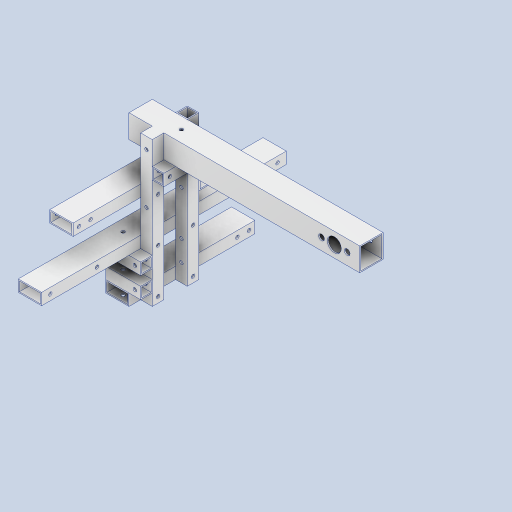
# Autodesk Inventor part: ballhand-v2-ASP-Base
Saved by Autodesk Inventor 2024 (Build 280153000, 153)
## iProperties
Created: 2024-03-16
Part Number: ballhand-v2-ASP-Base
Material: アルミニウム 6061
Document SubType Name: Modeling
Designer: haruy
Density: 2.7 g/cm^3
Appearance: アルミニウム - フラット
Author: haruy
Autodesk Inventor part; units mm, degrees
derived "ballhand-v2-Sketch-Base.ipt"
sketch "横から" plane through (0, 0, 0) normal (0, 0, 1) x (1, 0, 0)
  circle A0 centre (0, 0) radius 95
  line L0 (-321.6558, -95) -> (545.18, -95)
  line L1 (95, 81) -> (293, 81)
  line L2 (293, 81) -> (293, 61)
  line L3 (293, 61) -> (95, 61)
  line L4 (95, 61) -> (95, 81)
  line L5 (-52.5, 46.5) -> (145, 46.5)
  line L6 (145, 46.5) -> (145, 36.5)
  line L7 (145, 36.5) -> (-52.5, 36.5)
  line L8 (-52.5, 36.5) -> (-52.5, 46.5)
  line L9 (-52.5, -36.5) -> (145, -36.5)
  line L10 (145, -36.5) -> (145, -46.5)
  line L11 (145, -46.5) -> (-52.5, -46.5)
  line L12 (-52.5, -46.5) -> (-52.5, -36.5)
  line L13 (-50.5, 46.5) -> (-44.5, 46.5)
  line L14 (-44.5, 46.5) -> (-44.5, -46.5)
  line L15 (-44.5, -46.5) -> (-50.5, -46.5)
  line L16 (-50.5, -46.5) -> (-50.5, 46.5)
  line L17 (95, 5) -> (115, 5)
  line L18 (115, 5) -> (115, -5)
  line L19 (115, -5) -> (95, -5)
  line L20 (95, -5) -> (95, 5)
  line L21 (115, 4.5) -> (117.2, 4.5)
  line L22 (117.2, 4.5) -> (117.2, -4.5)
  line L23 (117.2, -4.5) -> (115, -4.5)
  line L24 (115, -4.5) -> (115, 4.5)
  line L25 (117.2, 10) -> (125, 10)
  line L26 (125, 10) -> (125, -10)
  line L27 (125, -10) -> (117.2, -10)
  line L28 (117.2, -10) -> (117.2, 10)
  line L29 (125, 46.5) -> (135, 46.5)
  line L30 (135, 46.5) -> (135, -46.5)
  line L31 (135, -46.5) -> (125, -46.5)
  line L32 (125, -46.5) -> (125, 46.5)
  line L33 (135, 36.5) -> (145, 36.5)
  line L34 (145, 36.5) -> (145, 26.5)
  line L35 (145, 26.5) -> (135, 26.5)
  line L36 (135, 26.5) -> (135, 36.5)
  line L37 (135, -36.5) -> (145, -36.5)
  line L38 (145, -36.5) -> (145, -26.5)
  line L39 (145, -26.5) -> (135, -26.5)
  line L40 (135, -26.5) -> (135, -36.5)
  line L41 (95, 33) -> (115, 33)
  line L42 (115, 33) -> (115, 43)
  line L43 (115, 43) -> (95, 43)
  line L44 (95, 43) -> (95, 33)
  line L45 (0, 0) -> (115, 0)
  line L46 (95, -33) -> (115, -33)
  line L47 (115, -43) -> (95, -43)
  line L48 (95, -43) -> (95, -33)
  line L49 (115, -33) -> (115, -43)
  line L50 (115, 81) -> (125, 81)
  line L51 (125, 81) -> (125, -43)
  line L52 (125, -43) -> (115, -43)
  line L53 (115, -43) -> (115, 81)
  circle A1 centre (105, 19) radius 2.5
  line L54 (125, 61) -> (135, 61)
  line L55 (135, 61) -> (135, 51)
  line L56 (135, 51) -> (125, 51)
  line L57 (125, 51) -> (125, 61)
  line L58 (95, 33) -> (125, 33)
  line L59 (125, 33) -> (125, 23)
  line L60 (125, 23) -> (95, 23)
  line L61 (95, 23) -> (95, 33)
  line L62 (95, -33) -> (125, -33)
  line L63 (125, -33) -> (125, -23)
  line L64 (125, -23) -> (95, -23)
  line L65 (95, -23) -> (95, -33)
  line L66 (95, -5) -> (125, -5)
  line L67 (125, -5) -> (125, -15)
  line L68 (125, -15) -> (95, -15)
  line L69 (95, -15) -> (95, -5)
  point P0 (120, 71)
  point P1 (271.25, 71)
  point P2 (260.25, 71)
  point P3 (282.25, 71)
  point P4 (120, 81)
  point P5 (120, 28)
  point P6 (120, -10)
  point P7 (120, -28)
  dimension "d1" = 10
  dimension "d2" = 10
  dimension "d3" = 30
  dimension "d4" = 10
  dimension "d7" = 30
  dimension "d8" = 10
  dimension "d9" = 30
  dimension "d10" = 10
  dimension "d11" = 21.75
  dimension "d12" = 11
  dimension "d13" = 11
  dimension "d14" = 10
  dimension "d15" = 10
  dimension "d16" = 10
  dimension "d17" = 5
  dimension "d18" = 10
  dimension "d19" = 5
  dimension "d20" = 5
  dimension "d21" = 5
  dimension "d22" = 5
  dimension "d23" = 5
  dimension "d24" = 5
  measures "d1" distance of L55.end L56.end
  measures "d2" distance of L54.end L55.end
  measures "d3" distance of L59.end L60.end
  measures "d4" distance of L58.end L59.end
  measures "d7" distance of L64.end L63.end
  measures "d8" distance of L63.end L62.end
  measures "d9" distance of L67.end L68.end
  measures "d10" distance of L66.end L67.end
  measures "d11" distance from line of point (271.25, 71) L2
  measures "d12" distance of point (271.25, 71) point (282.25, 71)
  measures "d13" distance of point (260.25, 71) point (271.25, 71)
  measures "d14" distance from line of point (260.25, 71) L1
  measures "d15" distance from line of point (271.25, 71) L1
  measures "d16" distance from line of point (282.25, 71) L1
  measures "d17" distance from line of L53 point (120, 71)
  measures "d18" distance of point (120, 71) point (120, 81)
  measures "d19" distance from line of point (120, 28) L32
  measures "d20" distance from line of L58 point (120, 28)
  measures "d21" distance from line of point (120, -10) L67
  measures "d22" distance from line of L66 point (120, -10)
  measures "d23" distance from line of point (120, -28) L51
  measures "d24" distance from line of L64 point (120, -28)
extrude "押し出し1" add sketch "横から" against normal blind 20 contours L53 L1 L51 L3 | L3 L4 L1 L53 | L51 L1 L2 L3
extrude "押し出し2" add sketch "横から" along normal blind 10 contours L18 L21 L22 L23 | L66 L28 L27 L32 L68 L53 | L18 L23 L28 L66 | L53 L60 L32 L25 L28 L21 L18 | L53 L3 L51 L5 | L5 L32 L7 L42 L53 | L7 L32 L58 L42 | L49 L62 L32 L9 | L9 L32 L52 L49 | L68 L32 L64 L53 | L66 L26 L27 L28 | L28 L22 L25 L26 L66 | L53 L58 L32 L60 | L53 L1 L51 L3 | L53 L64 L32 L62
ref_plane "作業平面1" through (293, 61, -20) normal (0, 0, -1) x (-1, 0, 0)
extrude "押し出し3" add sketch "横から" against normal blind 10 from surface at -20 separate body contours L18 L21 L22 L23 | L66 L28 L27 L32 L68 L53 | L18 L23 L28 L66 | L53 L60 L32 L25 L28 L21 L18 | L53 L3 L51 L5 | L5 L32 L7 L42 L53 | L7 L32 L58 L42 | L49 L62 L32 L9 | L9 L32 L52 L49 | L68 L32 L64 L53 | L66 L26 L27 L28 | L28 L22 L25 L26 L66 | L53 L58 L32 L60 | L53 L1 L51 L3 | L53 L64 L32 L62
extrude "押し出し4" add sketch "横から" along normal blind 10 and the other way blind 30 separate body contours L51 L3 L55 L56
extrude "押し出し5" add sketch "横から" along normal blind 95 and the other way blind 115 separate body contours L45 L18 L19 L20 | L20 L17 L18 L45
extrude "押し出し6" add sketch "横から" along normal blind 68 and the other way blind 40 separate body contours L44 L43 L42 L7 | L7 L42 L41 L44
extrude "押し出し7" add sketch "横から" along normal blind 20 and the other way blind 88 separate body contours L48 L46 L49 L9 | L9 L49 L47 L48
ref_plane "作業平面2" through (125, -43, -30) normal (0, 0, -1) x (-1, 0, 0)
extrude "押し出し8" add sketch "横から" against normal blind 10 from surface at -30 separate body contours L41 L53 L60 L61 | L53 L58 L32 L60
ref_plane "作業平面3" through (115, -43, 10) normal (0, 0, 1) x (1, 0, 0)
extrude "押し出し9" add sketch "横から" along normal blind 10 from surface at 10 separate body contours L65 L64 L53 L46 | L53 L64 L32 L62
extrude "押し出し10" add sketch "横から" along normal blind 10 from surface at 10 separate body contours L19 L53 L68 L69 | L66 L28 L27 L32 L68 L53 | L66 L26 L27 L28
shell "シェル1" thickness 1 removed faces 20 at (95, 74.3333, -13.3333) at (293, 67.6667, -6.6667) at (121.6667, 81, -23.3333) at (131.6667, 54.3333, -30) at (131.6667, 54.3333, 10) at (118.3333, -43, 3.3333) at (118.3333, -43, -23.3333) at (101.6667, -39.6667, 20) at (125, -29.6667, 13.3333) at (125, -8.3333, 16.6667) at (125, -13.3333, 13.3333) at (125, 26.3333, -33.3333) at (101.6667, -39.6667, -88) at (108.3333, -1.6667, -115) at (101.6667, 36.3333, -40) at (95, 29.6667, -33.3333) at (95, -26.3333, 13.3333) at (95, -8.3333, 13.3333) at (101.6667, 36.3333, 68) at (108.3333, -1.6667, 95) bodies 1 2 3 6 8 9 7 4 5
hole "穴1" at (120, 71, 0) at (120, -28, 0) at (120, -10, 0) at (120, 28, 0) direction (0, 0, -1) diameter 3 end through all both bodies 1 2 9 8 7
hole "穴2" at (271.25, 71, 0) direction (0, 0, -1) diameter 12 end through all bodies 1
hole "穴3" at (260.25, 71, 0) at (282.25, 71, 0) direction (0, 0, -1) diameter 5 end through all bodies 1
sketch "スケッチ3" plane through (135, 51, 10) normal (1, 0, 0) x (0, 0, -1)
  line L0 (40, 10) -> (0, 10) projected
  line L1 (40, 10) -> (40, 0) projected
  line L2 (0, 0) -> (0, 10) projected
  line L3 (0, 0) -> (40, 0) projected
  line L4 (30, -94) -> (30, 30) projected
  line L5 (50, -8) -> (-58, -8) projected
  line L6 (0, -94) -> (0, 30) projected
  line L7 (125, -46) -> (-85, -46) projected
  line L8 (40, -94) -> (30, -94) projected
  line L9 (98, -94) -> (-10, -94) projected
  point P0 (10, -51)
  point P1 (5, 5)
  point P2 (35, 5)
  point P3 (35, -13)
  point P4 (5, -13)
  point P5 (35, -51)
  point P6 (5, -51)
  point P7 (35, -89)
  point P8 (5, -89)
  dimension "d78" = 5
  dimension "d79" = 5
  dimension "d80" = 5
  dimension "d81" = 5
  dimension "d82" = 5
  dimension "d83" = 5
  dimension "d84" = 5
  dimension "d85" = 5
  dimension "d86" = 5
  dimension "d87" = 5
  dimension "d88" = 5
  dimension "d89" = 5
  dimension "d90" = 5
  dimension "d91" = 5
  dimension "d92" = 5
  dimension "d93" = 5
  measures "d78" distance from line of point (35, 5) L0
  measures "d79" distance from line of point (35, 5) L1
  measures "d80" distance from line of point (5, 5) L2
  measures "d81" distance from line of point (5, 5) L3
  measures "d82" distance from line of L4 point (35, -13)
  measures "d83" distance from line of L5 point (35, -13)
  measures "d84" distance from line of L6 point (5, -13)
  measures "d85" distance from line of point (5, -13) L5
  measures "d86" distance from line of L6 point (5, -51)
  measures "d87" distance from line of point (5, -51) L7
  measures "d88" distance from line of point (35, -51) L7
  measures "d89" distance from line of L4 point (35, -51)
  measures "d90" distance from line of L8 point (35, -89)
  measures "d91" distance from line of L4 point (35, -89)
  measures "d92" distance from line of L6 point (5, -89)
  measures "d93" distance from line of L9 point (5, -89)
hole "穴4" at (135, 56, 5) at (135, 56, -25) at (135, 38, -25) at (135, 38, 5) at (135, 0, -25) at (135, 0, 5) at (135, -38, -25) at (135, -38, 5) direction (-1, 0, 0) diameter 3 end through all bodies 3 5 1 2 4 6
sketch "スケッチ4" plane through (115, -5, 95) normal (1, 0, 0) x (0, 0, -1)
  line L0 (0, 0) -> (0, 10) projected
  line L1 (210, 0) -> (0, 0) projected
  line L2 (210, 10) -> (210, 0) projected
  line L3 (27, 38) -> (27, 48) projected
  line L4 (135, 48) -> (27, 48) projected
  line L5 (183, -28) -> (183, -38) projected
  line L6 (183, -28) -> (75, -28) projected
  point P0 (95, 5)
  point P1 (7.5, 5)
  point P2 (47.5, 5)
  point P3 (162.5, 5)
  point P4 (202.5, 5)
  point P5 (32, 43)
  point P6 (42, 43)
  point P7 (178, -33)
  point P8 (168, -33)
  dimension "d101" = 40
  dimension "d102" = 7.5
  dimension "d103" = 5
  dimension "d104" = 5
  dimension "d105" = 40
  dimension "d106" = 7.5
  dimension "d107" = 5
  dimension "d108" = 5
  dimension "d109" = 5
  dimension "d110" = 10
  dimension "d111" = 5
  dimension "d112" = 5
  dimension "d113" = 5
  dimension "d114" = 10
  dimension "d115" = 5
  dimension "d116" = 5
  measures "d101" distance of point (7.5, 5) point (47.5, 5)
  measures "d102" distance from line of L0 point (7.5, 5)
  measures "d103" distance from line of point (7.5, 5) L1
  measures "d104" distance from line of point (47.5, 5) L1
  measures "d105" distance of point (162.5, 5) point (202.5, 5)
  measures "d106" distance from line of point (202.5, 5) L2
  measures "d107" distance from line of point (162.5, 5) L1
  measures "d108" distance from line of point (202.5, 5) L1
  measures "d109" distance from line of L3 point (32, 43)
  measures "d110" distance of point (42, 43) point (32, 43)
  measures "d111" distance from line of L4 point (32, 43)
  measures "d112" distance from line of point (42, 43) L4
  measures "d113" distance from line of point (178, -33) L5
  measures "d114" distance of point (168, -33) point (178, -33)
  measures "d115" distance from line of point (168, -33) L6
  measures "d116" distance from line of point (178, -33) L6
hole "穴5" at (115, 0, 87.5) at (115, 0, 47.5) at (115, 0, -67.5) at (115, 0, -107.5) at (115, 38, 63) at (115, 38, 53) at (115, -38, -83) at (115, -38, -73) direction (-1, 0, 0) diameter 3 end through all bodies 4 5 6
sketch "スケッチ5" plane through (95, -43, 20) normal (0, -1, 0) x (1, 0, 0)
  line L0 (20, 0) -> (20, -108) projected
  line L1 (0, 0) -> (20, 0) projected
  point P0 (-95, -20)
  point P1 (10, -5)
  dimension "d124" = 10
  dimension "d125" = 5
  measures "d124" distance from line of point (10, -5) L0
  measures "d125" distance from line of point (10, -5) L1
hole "穴6" at (105, -43, 15) direction (0, 1, 0) diameter 3 end through all bodies 6 8 9 4
sketch "スケッチ6" plane through (125, 51, 10) normal (0, -1, 0) x (1, 0, 0)
  line L0 (10, 0) -> (10, -40) projected
  line L1 (168, -30) -> (-30, -30) projected
  point P0 (-125, -10)
  point P1 (5, -20)
  dimension "d133" = 5
  dimension "d134" = 10
  measures "d133" distance from line of point (5, -20) L0
  measures "d134" distance from line of point (5, -20) L1
hole "穴7" at (130, 51, -10) direction (0, 1, 0) diameter 3 end through all bodies 3 1
sketch "スケッチ7" plane through (95, 43, 68) normal (0, 1, 0) x (1, 0, 0)
  line L0 (0, 108) -> (20, 108) projected
  line L1 (20, 108) -> (20, 0) projected
  point P0 (-95, 68)
  point P1 (10, 103)
  dimension "d142" = 5
  dimension "d143" = 10
  measures "d142" distance from line of point (10, 103) L0
  measures "d143" distance from line of point (10, 103) L1
hole "穴8" at (105, 43, -35) direction (0, -1, 0) diameter 3 end through all bodies 5 7
equation "\"d15\" = d14"
equation "\"d16\" = d14"
equation "\"d22\" = d21"
equation "\"d79\" = d78"
equation "\"d104\" = d103"
equation "\"d116\" = d115"
